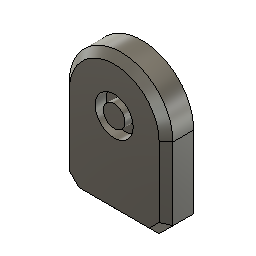
InvisibleHandle v4 (Autodesk Fusion 360 design; units mm, degrees)
Autodesk Fusion 360 part; units mm, degrees
note: some values were not read from the file. Set by a fixed rule: which sketch regions a step uses.
sketch "Sketch1" plane through (0, 0, 0) normal (0, 0, 1) x (1, 0, 0)
  circle A0 centre (0, 0) radius 7.5
  line L0 (-7.5, 0) -> (-7.5, -12.5)
  line L1 (-7.5, -12.5) -> (7.5, -12.5)
  line L2 (7.5, -12.5) -> (7.5, 0)
  circle A1 centre (0, 0) radius 4
  line L3 (-2, -12.5) -> (-2, -3.4641)
  line L4 (2, -3.4641) -> (2, -12.5)
  circle A2 centre (0, 0) radius 1.55
  circle A3 centre (0, 0) radius 2.75
  dimension "d1" = 15
  dimension "d2" = 20
  dimension "d3" = 8
  dimension "d4" = 4
  dimension "d5" = 3.1
  dimension "d6" = 5.5
  constraint coincident A0.centre A1.centre
  constraint coincident A0 L0.start
  constraint vertical L0
  constraint perpendicular L0 L1
  constraint coincident A0 L2.end
  constraint perpendicular L1 L2
  constraint tangent A0 L0
  constraint tangent A0 L2
  constraint coincident L1 L3.start
  constraint coincident A1 L3.end
  constraint perpendicular L1 L3
  constraint coincident A1 L4.start
  constraint coincident L1 L4.end
  constraint perpendicular L1 L4
  constraint equal L3 L4
  constraint concentric A1 A2
  constraint concentric A1 A3
  measures "d1" diameter of A0
  measures "d3" diameter of A1
  measures "d4" distance of L3 L4
  measures "d5" diameter of A2
  measures "d6" diameter of A3
extrude "Extrude1" add sketch "Sketch1" along normal blind 4 contours A0 A1 L3 L4 | A0 L1 L2 L4 | A0 L0 L1 L3 | A0 L1 L3 L4 | A0 A1 L3 L4 | A1 | A2 | A3
extrude "Extrude2" cut sketch "Sketch1" along normal blind 1.6 contours A0 L1 L3 L4 | A0 A1 L3 L4 | A1 | A2 | A3 picked at (0.436, -6.3069)
extrude "Extrude3" cut sketch "Sketch1" along normal through all contours A2
extrude "Extrude4" cut sketch "Sketch1" along normal up to surface (1.6 mm away) from surface at 2.4 contours A3
fillet "Fillet2" radius 5 2 edges at (2, -3.4641, 0.8) (-2, -3.4641, 0.8)
fillet "Fillet1" radius 0.8 5 edges at (2, -9.0784, 1.6) (2.286, -3.9902, 1.6) (0, 4, 1.6) (-2.286, -3.9902, 1.6) (-2, -9.0784, 1.6)
chamfer "Chamfer1" distance 2 angle 45 2 edges at (-7.5, -12.5, 2) (7.5, -12.5, 2)
chamfer "Chamfer2" distance 1 angle 45 6 edges at (-7.5, -5.25, 4) (7.5, -5.25, 4) (0, 7.5, 4) (0, -12.5, 4) (6.5, -11.5, 4) (-6.5, -11.5, 4)
cylinder "CylinderPrimitive1" add diameter 3.1 height -1.62 placed x (1, 0, 0) y (0, 1, 0) z (0, 0, 1) at (0, 0, 4)
equation "d12 = 4 mm - 1.6 mm"
named bodies: "Invisible Handle"
